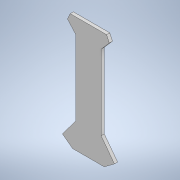
# Autodesk Inventor part: support_board_2
Saved by Autodesk Inventor 2020 (Build 240168000, 168)
## iProperties
Created: 2019-05-15
Part Number: support_board_2
Material: Generic
Document SubType Name: Modeling
Designer: psrob
Density: 1 g/cm^3
Appearance: Default
Author: psrob
Autodesk Inventor part; units mm, degrees
ref_plane "YZ Plane" through (0, 0, 0) normal (1, 0, 0) x (0, 1, 0)
ref_plane "XZ Plane" through (0, 0, 0) normal (0, 1, 0) x (-1, 0, 0)
ref_plane "XY Plane" through (0, 0, 0) normal (0, 0, 1) x (1, 0, 0)
sketch "Sketch1" plane through (0, 0, 0) normal (0, 0, 1) x (1, 0, 0)
  line L0 (39.9999, -8) -> (40, 85.1166) projected
  line L1 (40, 85.1166) -> (32.5, 95.1166) projected
  line L2 (32.5, 95.1166) -> (7.5, 95.1166) projected
  line L3 (7.5, 95.1166) -> (0, 85.1166) projected
  line L4 (0, 85.1166) -> (0, -8) projected
  line L5 (0, -8) -> (3.5294, -12) projected
  line L6 (3.5294, -12) -> (36.4705, -12) projected
  line L7 (36.4705, -12) -> (39.9999, -8) projected
  line L8 (25, -40) -> (28, -37) projected
  line L9 (28, -21.6) -> (28, -37) projected
  line L10 (39.9999, -8) -> (28, -21.6) projected
  line L11 (39.9999, 0) -> (39.9999, -8) projected
  line L12 (39.9999, 0) -> (20, 0) projected
  line L13 (20, 0) -> (20, -40) projected
  line L14 (25, -40) -> (20, -40) projected
  line L15 (18.0108, 135.1166) -> (18.0108, -64.8834)
  line L16 (15, -40) -> (12, -37) projected
  line L17 (15, -40) -> (20, -40) projected
  line L18 (20, 0) -> (20, -40) projected
  line L19 (0, 0) -> (20, 0) projected
  line L20 (0, 0) -> (0, -8) projected
  line L21 (0, -8) -> (12, -21.6) projected
  line L22 (12, -21.6) -> (12, -37) projected
  line L23 (40, -94.8834) -> (30, -84.8834) projected
  line L24 (40, -94.8834) -> (40, -84.8834) projected
  line L25 (25, -64.8834) -> (40, -84.8834) projected
  line L26 (25, -64.8834) -> (25, -54.8834) projected
  line L27 (25, -54.8834) -> (20, -54.8834) projected
  line L28 (20, -84.8834) -> (20, -54.8834) projected
  line L29 (30, -84.8834) -> (20, -84.8834) projected
  line L30 (0, -94.8834) -> (10, -84.8834) projected
  line L31 (10, -84.8834) -> (20, -84.8834) projected
  line L32 (20, -84.8834) -> (20, -54.8834) projected
  line L33 (15, -54.8834) -> (20, -54.8834) projected
  line L34 (15, -64.8834) -> (15, -54.8834) projected
  line L35 (15, -64.8834) -> (0, -84.8834) projected
  line L36 (0, -94.8834) -> (0, -84.8834) projected
  line L37 (30, -84.8834) -> (36.4, -80.0834)
  line L38 (10, -84.8834) -> (3.6, -80.0834)
  line L39 (15, -54.8834) -> (12, -37)
  line L40 (25, -54.8834) -> (28, -37)
  constraints: 10 end point, 2 perpendicular, 2 point on line, 1 vertical, 2 other
extrude "Extrusion1" add sketch "Sketch1" along normal blind 2 contours L10 L9 L8 L14 L13 L6 | L13 L17 L15 L6 | L15 L17 L16 L22 L21 L6 | L14 L8 L40 L27 L33 L15 L17 | L15 L33 L39 L16 L17 | L26 L25 L37 L29 L28 L27 | L33 L28 L31 L38 L35 L34
chamfer "Chamfer1" distance 5 angle 45 2 edges at (3.5294, -12, 1) (36.4705, -12, 1)
sketch "Sketch2" plane through (0, 0, 2) normal (0, 0, 1) x (1, 0, 0)
  line L0 (31.4705, -12) -> (33.1624, -15.7492) projected
  line L1 (31.4705, -12) -> (8.5294, -12) projected
  line L2 (6.8375, -15.7492) -> (8.5294, -12) projected
  line L3 (6.8375, -15.7492) -> (12, -21.6) projected
  line L4 (12, -21.6) -> (12, -37) projected
  line L5 (12, -37) -> (15, -54.8834) projected
  line L6 (15, -54.8834) -> (15, -64.8834) projected
  line L7 (15, -64.8834) -> (3.6, -80.0834) projected
  line L8 (3.6, -80.0834) -> (10, -84.8834) projected
  line L9 (10, -84.8834) -> (30, -84.8834) projected
  line L10 (30, -84.8834) -> (36.4, -80.0834) projected
  line L11 (36.4, -80.0834) -> (25, -64.8834) projected
  line L12 (25, -64.8834) -> (25, -54.8834) projected
  line L13 (25, -54.8834) -> (28, -37) projected
  line L14 (28, -37) -> (28, -21.6) projected
  line L15 (28, -21.6) -> (33.1624, -15.7492) projected
  line L16 (12, -37) -> (12, -68.8835)
  line L17 (15, -64.8834) -> (3.6, -80.0834) projected
  line L18 (25, -54.8834) -> (28, -37) projected
  line L19 (28, -37) -> (28, -68.8834)
  line L20 (36.4, -80.0834) -> (25, -64.8834) projected
  point P0 (0, 0)
  constraints: 4 end point, 2 point on line, 1 parallel, 1 vertical
extrude "Extrusion2" add sketch "Sketch2" against normal blind 2 contours L19 L11 L12 L13 | L5 L6 L7 L16
body "Solid1"
